Autodesk Inventor part; units mm, degrees
(part 3 of 6)
  line L865 (0, -261.6424) -> (21.9118, -283.5542) projected
  line L866 (149.4183, -199.8451) -> (131.1117, -181.5385) projected
  line L867 (131.1117, -181.5385) -> (153.0236, -159.6267) projected
  line L868 (153.0236, -159.6267) -> (165.1681, -171.7713) projected
  arc A19 (165.1681, -171.7713) -> (149.4183, -199.8451) centre (222.25, -222.25) ccw projected
  arc A20 (222.25, -146.05) -> (217.4573, -146.2009) centre (222.25, -222.25) ccw projected
  line L869 (217.4573, -146.2009) -> (229.5353, -134.1228) projected
  line L870 (229.5353, -134.1228) -> (241.4626, -146.05) projected
  line L871 (241.4626, -146.05) -> (222.25, -146.05) projected
  line L872 (280.5432, -75.9307) -> (258.6314, -54.0189) projected
  line L873 (258.6314, -54.0189) -> (280.5432, -32.1071) projected
  line L874 (280.5432, -32.1071) -> (298.45, -50.0139) projected
  line L875 (298.45, -50.0139) -> (298.45, -58.0239) projected
  line L876 (298.45, -58.0239) -> (280.5432, -75.9307) projected
  line L877 (284.1353, -28.515) -> (298.45, -14.2003) projected
  line L878 (298.45, -14.2003) -> (298.45, -42.8297) projected
  line L879 (298.45, -42.8297) -> (284.1353, -28.515) projected
  line L880 (204.0314, -57.611) -> (225.9432, -79.5228) projected
  line L881 (225.9432, -79.5228) -> (204.0314, -101.4346) projected
  line L882 (204.0314, -101.4346) -> (182.1196, -79.5228) projected
  line L883 (182.1196, -79.5228) -> (204.0314, -57.611) projected
  line L884 (102.0157, -203.4504) -> (80.1039, -181.5385) projected
  line L885 (80.1039, -181.5385) -> (102.0157, -159.6267) projected
  line L886 (102.0157, -159.6267) -> (123.9275, -181.5385) projected
  line L887 (123.9275, -181.5385) -> (102.0157, -203.4504) projected
  line L888 (36.8076, -298.45) -> (14.2003, -298.45) projected
  line L889 (14.2003, -298.45) -> (25.5039, -287.1463) projected
  line L890 (25.5039, -287.1463) -> (36.8076, -298.45) projected
  line L891 (94.9996, -298.45) -> (80.1039, -283.5542) projected
  line L892 (80.1039, -283.5542) -> (102.0157, -261.6424) projected
  line L893 (102.0157, -261.6424) -> (123.9275, -283.5542) projected
  line L894 (123.9275, -283.5542) -> (109.0318, -298.45) projected
  line L895 (109.0318, -298.45) -> (94.9996, -298.45) projected
  line L896 (-65.2081, -298.45) -> (-87.8154, -298.45) projected
  line L897 (-87.8154, -298.45) -> (-76.5118, -287.1463) projected
  line L898 (-76.5118, -287.1463) -> (-65.2081, -298.45) projected
  line L899 (-29.096, -283.5542) -> (-43.9918, -298.45) projected
  line L900 (-43.9918, -298.45) -> (-58.0239, -298.45) projected
  line L901 (-58.0239, -298.45) -> (-72.9197, -283.5542) projected
  line L902 (-72.9197, -283.5542) -> (-51.0079, -261.6424) projected
  line L903 (-51.0079, -261.6424) -> (-29.096, -283.5542) projected
  line L904 (-51.0079, -210.6346) -> (-29.096, -232.5464) projected
  line L905 (-29.096, -232.5464) -> (-51.0079, -254.4582) projected
  line L906 (-51.0079, -254.4582) -> (-72.9197, -232.5464) projected
  line L907 (-72.9197, -232.5464) -> (-51.0079, -210.6346) projected
  line L908 (-146.05, -247.4846) -> (-146.05, -222.25) projected
  arc A21 (-146.05, -222.25) -> (-146.2009, -217.4573) centre (-222.25, -222.25) ccw projected
  line L909 (-146.2009, -217.4573) -> (-131.1117, -232.5464) projected
  line L910 (-131.1117, -232.5464) -> (-146.05, -247.4846) projected
  line L911 (-51.0079, -152.4425) -> (-72.9197, -130.5307) projected
  line L912 (-72.9197, -130.5307) -> (-51.0079, -108.6189) projected
  line L913 (-51.0079, -108.6189) -> (-29.096, -130.5307) projected
  line L914 (-29.096, -130.5307) -> (-51.0079, -152.4425) projected
  line L915 (0, -101.4346) -> (-21.9118, -79.5228) projected
  line L916 (-21.9118, -79.5228) -> (0, -57.611) projected
  line L917 (0, -57.611) -> (21.9118, -79.5228) projected
  line L918 (21.9118, -79.5228) -> (0, -101.4346) projected
  line L919 (51.0079, -159.6267) -> (72.9197, -181.5385) projected
  line L920 (72.9197, -181.5385) -> (51.0079, -203.4504) projected
  line L921 (51.0079, -203.4504) -> (29.096, -181.5385) projected
  line L922 (29.096, -181.5385) -> (51.0079, -159.6267) projected
  line L923 (-76.5118, -134.1228) -> (-54.6, -156.0346) projected
  line L924 (-54.6, -156.0346) -> (-76.5118, -177.9464) projected
  line L925 (-76.5118, -177.9464) -> (-98.4236, -156.0346) projected
  line L926 (-98.4236, -156.0346) -> (-76.5118, -134.1228) projected
  line L927 (-153.0236, -108.6189) -> (-131.1117, -130.5307) projected
  line L928 (-131.1117, -130.5307) -> (-153.0236, -152.4425) projected
  line L929 (-153.0236, -152.4425) -> (-174.9354, -130.5307) projected
  line L930 (-174.9354, -130.5307) -> (-153.0236, -108.6189) projected
  line L931 (-178.5275, -83.1149) -> (-156.6157, -105.0267) projected
  line L932 (-156.6157, -105.0267) -> (-178.5275, -126.9386) projected
  line L933 (-178.5275, -126.9386) -> (-200.4393, -105.0267) projected
  line L934 (-200.4393, -105.0267) -> (-178.5275, -83.1149) projected
  line L935 (-233.1274, -79.5228) -> (-255.0393, -101.4346) projected
  line L936 (-255.0393, -101.4346) -> (-276.9511, -79.5228) projected
  line L937 (-276.9511, -79.5228) -> (-255.0393, -57.611) projected
  line L938 (-255.0393, -57.611) -> (-233.1274, -79.5228) projected
  line L939 (-258.6314, -105.0267) -> (-280.5432, -126.9386) projected
  line L940 (-280.5432, -126.9386) -> (-298.45, -109.0318) projected
  line L941 (-298.45, -109.0318) -> (-298.45, -101.0217) projected
  line L942 (-298.45, -101.0217) -> (-280.5432, -83.1149) projected
  line L943 (-280.5432, -83.1149) -> (-258.6314, -105.0267) projected
  circle A22 centre (-304.8, 0) radius 1.9939 projected
  circle A23 centre (-304.8, -44.45) radius 1.9939 projected
  circle A24 centre (-88.9, -304.8) radius 1.9939 projected
  circle A25 centre (88.9, -304.8) radius 1.9939 projected
  circle A26 centre (304.8, -44.45) radius 1.9939 projected
  circle A27 centre (304.8, 133.35) radius 1.9939 projected
  circle A28 centre (0, 304.8) radius 1.9939 projected
  circle A29 centre (-133.35, 304.8) radius 1.9939 projected
  circle A30 centre (44.45, 304.8) radius 1.9939 projected
  circle A31 centre (304.8, 88.9) radius 1.9939 projected
  circle A32 centre (304.8, -88.9) radius 1.9939 projected
  circle A33 centre (44.45, -304.8) radius 1.9939 projected
  circle A34 centre (-133.35, -304.8) radius 1.9939 projected
  circle A35 centre (-304.8, 44.45) radius 1.9939 projected
  circle A36 centre (-304.8, 133.35) radius 1.9939 projected
  circle A37 centre (-304.8, -88.9) radius 1.9939 projected
  circle A38 centre (-44.45, -304.8) radius 1.9939 projected
  circle A39 centre (133.35, -304.8) radius 1.9939 projected
  circle A40 centre (133.35, 304.8) radius 1.9939 projected
  circle A41 centre (-44.45, 304.8) radius 1.9939 projected
  circle A42 centre (-88.9, 304.8) radius 1.9939 projected
  circle A43 centre (88.9, 304.8) radius 1.9939 projected
  circle A44 centre (304.8, 44.45) radius 1.9939 projected
  circle A45 centre (304.8, -133.35) radius 1.9939 projected
  circle A46 centre (0, -304.8) radius 1.9939 projected
  circle A47 centre (-304.8, -133.35) radius 1.9939 projected
  circle A48 centre (-304.8, 88.9) radius 1.9939 projected
  line L944 (-311.15, -158.75) -> (-222.25, -158.75) projected
  arc A49 (-158.75, -222.25) -> (-222.25, -158.75) centre (-222.25, -222.25) ccw projected
  line L945 (-158.75, -222.25) -> (-158.75, -311.15) projected
  line L946 (-158.75, -311.15) -> (158.75, -311.15) projected
  line L947 (158.75, -311.15) -> (158.75, -222.25) projected
  arc A50 (222.25, -158.75) -> (158.75, -222.25) centre (222.25, -222.25) ccw projected
  line L948 (222.25, -158.75) -> (311.15, -158.75) projected
  line L949 (311.15, -158.75) -> (311.15, 158.75) projected
  line L950 (311.15, 158.75) -> (222.25, 158.75) projected
  arc A51 (158.75, 222.25) -> (222.25, 158.75) centre (222.25, 222.25) ccw projected
  line L951 (158.75, 222.25) -> (158.75, 311.15) projected
  line L952 (158.75, 311.15) -> (-158.75, 311.15) projected
  line L953 (-158.75, 311.15) -> (-158.75, 222.25) projected
  arc A52 (-222.25, 158.75) -> (-158.75, 222.25) centre (-222.25, 222.25) ccw projected
  line L954 (-222.25, 158.75) -> (-311.15, 158.75) projected
  line L955 (-311.15, 158.75) -> (-311.15, -158.75) projected
  line L956 (0, -311.15) -> (0, 311.15)
  line L957 (-311.15, 158.75) -> (-311.15, -158.75) projected
  line L958 (-311.15, 0) -> (311.15, 0)
  line L959 (81.1911, -89.119) -> (-81.1911, -89.119)
  line L960 (-81.1911, 90.2812) -> (81.1911, 90.2812)
  line L961 (84.3661, -89.119) -> (-84.3661, 90.2812) construction
  line L962 (-84.3661, -89.119) -> (84.3661, 90.2812) construction
  line L963 (88.0954, 51.4208) -> (87.5411, 51.4208)
  line L964 (73.7326, 23.3058) -> (73.7326, 21.68)
  line L965 (-84.3661, 54.5958) -> (-84.3661, 87.1062)
  line L966 (-84.3661, -85.944) -> (-84.3661, -53.4337)
  line L967 (84.3661, -53.4337) -> (84.3661, -85.944)
  line L968 (84.3661, 87.1062) -> (84.3661, 54.5958)
  arc A53 (81.1911, -89.119) -> (84.3661, -85.944) centre (81.1911, -85.944) ccw
  arc A54 (-84.3661, -85.944) -> (-81.1911, -89.119) centre (-81.1911, -85.944) ccw
  arc A55 (-81.1911, 90.2812) -> (-84.3661, 87.1062) centre (-81.1911, 87.1062) ccw
  arc A56 (84.3661, 87.1062) -> (81.1911, 90.2812) centre (81.1911, 87.1062) ccw
  arc A57 (87.5411, -50.2587) -> (84.3661, -53.4337) centre (87.5411, -53.4337) ccw
  arc A58 (84.3661, 54.5958) -> (87.5411, 51.4208) centre (87.5411, 54.5958) ccw
  line L969 (91.2704, -47.0837) -> (91.2704, 48.2458)
  line L970 (87.5411, -50.2587) -> (88.0954, -50.2587)
  line L971 (94.6634, -50.2587) -> (94.9996, -50.2587)
  arc A59 (88.0954, -50.2587) -> (91.2704, -47.0837) centre (88.0954, -47.0837) ccw
  arc A60 (91.2704, 48.2458) -> (88.0954, 51.4208) centre (88.0954, 48.2458) ccw
  line L972 (-94.6634, -50.2587) -> (-94.9996, -50.2587)
  arc A61 (-84.3661, -53.4337) -> (-87.5411, -50.2587) centre (-87.5411, -53.4337) ccw
  arc A62 (-84.3661, -53.4337) -> (-87.5411, -50.2587) centre (-87.5411, -53.4337) ccw
  arc A63 (-87.5411, 51.4208) -> (-84.3661, 54.5958) centre (-87.5411, 54.5958) ccw
  line L973 (-91.2704, -47.0837) -> (-91.2704, 48.2458)
  arc A64 (-91.2704, -47.0837) -> (-88.0954, -50.2587) centre (-88.0954, -47.0837) ccw
  arc A65 (-88.0954, 51.4208) -> (-91.2704, 48.2458) centre (-88.0954, 48.2458) ccw
  line L974 (-88.0954, -50.2587) -> (-87.5411, -50.2587)
  line L975 (-87.5411, 51.4208) -> (-88.0954, 51.4208)
  line L976 (-87.9035, -53.4337) -> (-87.9035, -85.944)
  arc A66 (-87.9035, -85.944) -> (-81.1911, -92.6564) centre (-81.1911, -85.944) ccw
  line L977 (-81.1911, -92.6564) -> (81.1911, -92.6564)
  arc A67 (81.1911, -92.6564) -> (87.9035, -85.944) centre (81.1911, -85.944) ccw
  line L978 (87.9035, -85.944) -> (87.9035, -53.7961)
  line L979 (87.9035, -53.7961) -> (88.0954, -53.7961)
  arc A68 (88.0954, -53.7961) -> (94.8078, -47.0837) centre (88.0954, -47.0837) ccw
  line L980 (94.8078, -47.0837) -> (94.8078, 48.2458)
  arc A69 (94.8078, 48.2458) -> (88.0954, 54.9582) centre (88.0954, 48.2458) ccw
  line L981 (88.0954, 54.9582) -> (87.9035, 54.9582)
  line L982 (87.9035, 54.9582) -> (87.9035, 87.1062)
  arc A70 (87.9035, 87.1062) -> (81.1911, 93.8186) centre (81.1911, 87.1062) ccw
  line L983 (81.1911, 93.8186) -> (-81.1911, 93.8186)
  arc A71 (-81.1911, 93.8186) -> (-87.9035, 87.1062) centre (-81.1911, 87.1062) ccw
  line L984 (-87.9035, 87.1062) -> (-87.9035, 54.9582)
  line L985 (-87.9035, 54.9582) -> (-88.0954, 54.9582)
  arc A72 (-88.0954, 54.9582) -> (-94.8078, 48.2458) centre (-88.0954, 48.2458) ccw
  line L986 (-94.8078, 48.2458) -> (-94.8078, -47.0837)
  arc A73 (-94.8078, -47.0837) -> (-88.0954, -53.7961) centre (-88.0954, -47.0837) ccw
  line L987 (-88.0954, -53.7961) -> (-87.5411, -53.7961)
  point P0 (0, 0)
  point P1 (84.3661, 0.5811)
  point P2 (84.3661, -50.2587)
  point P3 (-84.3661, -50.2587)
  point P4 (-84.3661, 51.4208)
  point P5 (84.3661, 51.4208)
  point P6 (-31.508, -89.119)
  point P7 (-19.4998, -89.119)
  point P8 (-84.3661, -75.2606)
  point P9 (-84.3661, -83.785)
  point P10 (-82.3116, -88.9147)
  point P11 (-70.5077, -89.119)
  point P12 (-91.2704, -17.3485)
  point P13 (-91.2704, -39.6815)
  point P14 (-91.2704, -46.8657)
  point P15 (-84.3661, -68.0764)
  point P16 (-63.3235, -89.119)
  point P17 (-38.6922, -89.119)
  point P18 (-91.2704, -10.1643)
  point P19 (-57.611, 0)
  point P20 (-44.4047, 0)
  point P21 (-6.6031, 0)
  point P22 (0, 0)
  point P23 (0, -50.4268)
  point P24 (0, -57.611)
  point P25 (0, -57.611)
  point P26 (12.3156, -89.119)
  point P27 (-12.3156, -89.119)
  point P28 (0, -89.119)
  point P29 (52.6018, 93.8186)
  point P30 (49.4139, 93.8186)
  point P31 (-87.9035, -53.7961)
  dimension "d116" = 168.7322
  dimension "d117" = 179.4002
  dimension "d120" = 3.175
  dimension "d121" = 3.175
  dimension "d122" = 3.175
  constraints: 62 end point, 42 point on circle, 21 centre point, 18 tangent, 16 point on line, 13 parallel, 13 symmetric about line, 6 equal radius, 6 midpoint, 4 horizontal, 4 perpendicular, 23 other
  measures "d116" distance of L961.end L962.end
  measures "d117" distance of L962.start L961.end
  measures "d120" radius of A53
  measures "d121" radius of A59
  measures "d122" radius of A61
extrude "Extrusion13" add sketch "Sketch12" against normal up to surface (3.175 mm away) contours L977 L183 L959 L915 | L915 L959 L956 L977 | L977 L956 L959 L918 | L918 L959 L487 L977 | L977 L186 L959 L183 | L487 L959 L488 L977 | L977 L662 L959 L186 | L488 L959 L21 L977 | L977 L663 L959 L662 | L21 L959 L24 L977 | L977 L198 L959 L663 | L24 L959 L321 L977 | L977 A66 L197 A54 L959 L198 | L321 L959 A53 L322 A67 L977 | A66 L258 L966 A54 L197 | L322 A53 L967 L832 A67 | A66 L976 L257 L966 L258 | L832 L967 L833 L978 A67 | L960 L751 L983 L956 | L956 L983 L748 L960 | L973 L187 L986 L958 | L958 L986 L188 L973 | L969 L352 L980 L958 | L958 L980 L353 L969 | L257 L976 L667 L966 | L967 L571 L978 L833 | L748 L983 L129 L960 | L960 L275 L983 L751 | L188 L986 L652 L973 | L973 L736 L986 L187 | L969 L574 L980 L352 | L353 L980 L99 L969 | L667 L976 L987 A73 L668 L973 A64 L974 A61 L966 | L967 A57 L970 A59 L969 L570 A68 L979 L978 L571 | L129 L983 L128 L960 | L960 L276 L983 L275 | L652 L986 L651 L973 | L973 L737 L986 L736 | L969 L575 L980 L574 | L99 L980 L98 L969 | L128 L983 L115 L960 | L960 L178 L983 L276 | L651 L986 L753 L973 | L973 L668 A73 L986 L737 | L969 L585 L980 L575 | L98 L980 A68 L570 L969 | L115 L983 L112 L960 | L960 L177 L983 L178 | L753 L986 A72 L985 L984 L754 L965 A63 L975 A65 L973 | L969 A60 L963 A58 L968 L584 L982 L981 A69 L980 L585 | L115 L112 L983 | L112 L983 L822 L960 | L960 L165 L983 L177 | L822 L983 A70 L821 L968 A56 L960 | L960 A55 L965 L166 A71 L983 L165 | L984 L172 L965 L754 | L584 L968 L350 L982 | L821 A70 L982 L351 L968 | L965 L171 L984 A71 L166 | L984 L171 L965 L172 | L350 L968 L351 L982
sketch "Sketch13" plane through (0, 3.175, 0) normal (0, 1, 0) x (1, 0, 0)
  line L0 (-70.5077, -89.119) -> (-81.1911, -89.119) projected
  arc A0 (-82.3116, -88.9147) -> (-81.1911, -89.119) centre (-81.1911, -85.944) ccw projected
  line L1 (-84.3661, -83.785) -> (-84.3661, -75.2606) projected
  line L2 (81.1911, -89.119) -> (70.5077, -89.119) projected
  line L3 (84.3661, -75.2606) -> (84.3661, -83.785) projected
  line L4 (-78.0506, -89.119) -> (-81.1911, -89.119)
  line L5 (-84.3661, -80.2772) -> (-84.3661, -85.944)
  line L6 (63.3235, 90.2812) -> (81.1911, 90.2812) projected
  line L7 (84.3661, 77.763) -> (84.3661, 69.2385) projected
  line L8 (84.3661, 87.1062) -> (84.3661, 84.9472) projected
  line L9 (78.1452, 90.2812) -> (81.1911, 90.2812)
  line L10 (84.3661, 87.1062) -> (84.3661, 85.7634)
  line L11 (81.1911, 90.2812) -> (-81.1911, 90.2812)
  line L12 (-81.1911, -89.119) -> (81.1911, -89.119)
  arc A1 (-84.3661, -85.944) -> (-81.1911, -89.119) centre (-81.1911, -85.944) ccw
  arc A2 (81.1911, -89.119) -> (84.3661, -85.944) centre (81.1911, -85.944) ccw
  arc A3 (-84.3661, -85.944) -> (-81.1911, -89.119) centre (-81.1911, -85.944) ccw
  arc A4 (-81.1911, 90.2812) -> (-84.3661, 87.1062) centre (-81.1911, 87.1062) ccw
  arc A5 (84.3661, 87.1062) -> (81.1911, 90.2812) centre (81.1911, 87.1062) ccw
  arc A6 (84.3661, 87.1062) -> (81.1911, 90.2812) centre (81.1911, 87.1062) ccw
  arc A7 (87.5411, -50.2587) -> (84.3661, -53.4337) centre (87.5411, -53.4337) ccw projected
  arc A8 (88.0954, -50.2587) -> (91.2704, -47.0837) centre (88.0954, -47.0837) ccw projected
  line L13 (91.2704, -17.3485) -> (91.2704, -39.6815) projected
  arc A9 (84.3661, 54.5958) -> (87.5411, 51.4208) centre (87.5411, 54.5958) ccw projected
  arc A10 (91.2704, 48.2458) -> (88.0954, 51.4208) centre (88.0954, 48.2458) ccw projected
  line L14 (91.2704, 48.2458) -> (91.2704, 40.8436) projected
  line L15 (91.2704, -39.6815) -> (91.2704, -17.3485) projected
  line L16 (84.3661, -85.944) -> (84.3661, -53.4337)
  line L17 (84.3661, 54.5958) -> (84.3661, 87.1062)
  arc A11 (-84.3661, -53.4337) -> (-87.5411, -50.2587) centre (-87.5411, -53.4337) ccw projected
  arc A12 (-91.2704, -47.0837) -> (-88.0954, -50.2587) centre (-88.0954, -47.0837) ccw projected
  line L18 (-87.5411, -50.2587) -> (-88.0954, -50.2587) projected
  line L19 (-91.2704, -47.0837) -> (-91.2704, -46.8657) projected
  arc A13 (-87.5411, 51.4208) -> (-84.3661, 54.5958) centre (-87.5411, 54.5958) ccw projected
  arc A14 (-88.0954, 51.4208) -> (-91.2704, 48.2458) centre (-88.0954, 48.2458) ccw projected
  line L20 (-91.2704, 40.8436) -> (-91.2704, 48.2458) projected
  line L21 (-91.2704, -46.8657) -> (-91.2704, 40.8436)
  line L22 (-84.3661, 87.1062) -> (-84.3661, 54.5958)
  line L23 (-84.3661, -53.4337) -> (-84.3661, -85.944)
  line L24 (91.2704, -46.8657) -> (91.2704, -47.0837) projected
  line L25 (91.2704, 40.8436) -> (91.2704, 48.2458) projected
  line L26 (91.2704, 44.2779) -> (91.2704, -46.8657)
  line L27 (87.5411, 51.4208) -> (88.0954, 51.4208) projected
  line L28 (88.0954, -50.2587) -> (87.5411, -50.2587) projected
  line L29 (-88.0954, 51.4208) -> (-87.5411, 51.4208) projected
  point P0 (0, 0)
  point P1 (-85.248, -89.119)
  point P2 (-84.3661, -89.119)
  point P3 (84.3661, 90.2812)
  point P4 (-82.3116, -88.9147)
  dimension "d125" = 3.175
  constraints: 24 end point, 16 point on circle, 16 tangent, 15 point on line, 6 centre point, 5 equal radius, 5 parallel, 2 collinear, 2 perpendicular, 1 horizontal
  measures "d125" radius of A1
extrude "Extrusion14" cut sketch "Sketch13" against normal blind 80.9625
sketch "Sketch14" plane through (0, 3.175, 0) normal (0, 1, 0) x (1, 0, 0)
  arc A0 (-84.9214, -91.5245) -> (-81.1911, -92.6564) centre (-81.1911, -85.944) ccw projected
  line L0 (-81.1911, -92.6564) -> (-66.9703, -92.6564) projected
  line L1 (-79.3946, -92.6564) -> (-81.1979, -92.6564)
  line L2 (-81.1911, 90.2812) -> (81.1911, 90.2812) projected
  line L3 (87.9035, 65.7011) -> (87.9035, 81.3004) projected
  line L4 (81.1911, 93.8186) -> (59.7861, 93.8186) projected
  line L5 (87.9035, 76.3407) -> (87.9035, 87.113)
  line L6 (81.1979, 93.8186) -> (78.2104, 93.8186)
  line L7 (-81.1979, -92.6564) -> (81.1979, -92.6564)
  line L8 (81.1979, 93.8186) -> (-81.1979, 93.8186)
  line L9 (-87.9035, 87.113) -> (-87.9035, 54.9582)
  line L10 (-94.8078, -13.8111) -> (-94.8078, -43.2189) projected
  line L11 (-94.8078, -41.8566) -> (-94.8078, -47.0905)
  line L12 (-88.1022, -53.7961) -> (-88.0954, -53.7961)
  arc A1 (-94.2247, -49.82) -> (-88.0954, -53.7961) centre (-88.0954, -47.0837) ccw projected
  arc A2 (-94.8078, -47.0905) -> (-88.1022, -53.7961) centre (-88.1022, -47.0905) ccw
  arc A3 (-88.0954, 54.9582) -> (-94.8078, 48.2458) centre (-88.0954, 48.2458) ccw projected
  line L13 (-87.9035, 54.9582) -> (-88.0954, 54.9582) projected
  line L14 (-94.8078, 48.2458) -> (-94.8078, 44.381) projected
  line L15 (-94.8078, 46.3134) -> (-94.8078, -47.0905)
  arc A4 (-87.9035, -85.9508) -> (-81.1979, -92.6564) centre (-81.1979, -85.9508) ccw
  arc A5 (-81.1979, 93.8186) -> (-87.9035, 87.113) centre (-81.1979, 87.113) ccw
  arc A6 (87.9035, 87.113) -> (81.1979, 93.8186) centre (81.1979, 87.113) ccw
  line L16 (87.9035, -85.9508) -> (87.9035, -53.7961)
  line L17 (87.9035, 54.9582) -> (87.9035, 87.113)
  line L18 (94.8078, -43.2189) -> (94.8078, -13.8111) projected
  line L19 (94.8078, 44.381) -> (94.8078, 48.2458) projected
  arc A7 (94.8078, 48.2458) -> (88.0954, 54.9582) centre (88.0954, 48.2458) ccw projected
  line L20 (88.0954, 54.9582) -> (87.9035, 54.9582) projected
  arc A8 (88.0954, -53.7961) -> (94.2247, -49.82) centre (88.0954, -47.0837) ccw projected
  line L21 (87.9035, -53.7961) -> (88.0954, -53.7961) projected
  line L22 (94.8078, 46.3134) -> (94.8078, -47.0905)
  line L23 (88.1022, -53.7961) -> (88.0954, -53.7961)
  arc A9 (88.1022, -53.7961) -> (94.8078, -47.0905) centre (88.1022, -47.0905) ccw
  arc A10 (81.1979, -92.6564) -> (87.9035, -85.9508) centre (81.1979, -85.9508) ccw
  line L24 (81.1979, -92.6564) -> (-81.1979, -92.6564)
  line L25 (-87.9035, -85.9508) -> (-87.9035, -53.7961)
  line L26 (-94.8078, -47.0905) -> (-94.8078, 46.3134)
  line L27 (-87.9035, 58.5169) -> (-87.9035, 54.9582) projected
  line L28 (-87.9035, 54.9582) -> (-87.9035, 87.113)
  line L29 (-81.1979, 93.8186) -> (81.1979, 93.8186)
  line L30 (87.9035, 87.113) -> (87.9035, 54.9582)
  line L31 (-81.1979, -102.0798) -> (81.1979, -102.0798)
  arc A11 (-97.3269, -85.9508) -> (-81.1979, -102.0798) centre (-81.1979, -85.9508) ccw
  line L32 (-88.0954, -53.7961) -> (-87.9035, -53.7961) projected
  line L33 (-87.9035, -53.7961) -> (-88.0954, -53.7961)
  line L34 (97.325, -60.3125) -> (97.325, -85.9508)
  arc A12 (81.1979, -102.0779) -> (97.325, -85.9508) centre (81.1979, -85.9508) ccw
  line L35 (104.223, 44.3468) -> (104.223, -47.0905)
  arc A13 (97.325, -60.3125) -> (104.223, -47.0905) centre (88.1022, -47.0905) ccw
  line L36 (88.1022, -63.2113) -> (88.0954, -63.2113)
  line L37 (87.9035, 64.3816) -> (88.0954, 64.3816)
  arc A14 (104.2312, 48.2458) -> (97.3269, 61.4799) centre (88.0954, 48.2458) ccw
  line L38 (104.2312, 48.2458) -> (104.2312, 44.381)
  line L39 (97.3269, 61.4799) -> (97.3269, 87.113)
  arc A15 (97.3269, 87.113) -> (81.1979, 103.242) centre (81.1979, 87.113) ccw
  line L40 (81.1979, 103.242) -> (-81.1979, 103.242)
  arc A16 (-81.1979, 103.242) -> (-97.3269, 87.113) centre (-81.1979, 87.113) ccw
  line L41 (-97.3269, 87.113) -> (-97.3269, 61.4799)
  line L42 (-94.8078, -47.0905) -> (-94.8078, 46.3134)
  line L43 (-104.2312, -47.0905) -> (-104.2312, 46.3134)
  line L44 (-104.2312, 46.3134) -> (-104.2312, 48.2458)
  arc A17 (-94.8078, -47.0905) -> (-88.0988, -53.7961) centre (-88.1022, -47.0905) ccw
  arc A18 (-104.2312, -47.0905) -> (-97.3269, -60.3211) centre (-88.1022, -47.0905) ccw
  line L45 (-97.3269, -85.9508) -> (-97.3269, -60.3211)
  arc A19 (-97.3269, 61.4799) -> (-104.2312, 48.2458) centre (-88.0954, 48.2458) ccw
  arc A20 (87.5411, -50.2587) -> (84.3661, -53.4337) centre (87.5411, -53.4337) ccw projected
  line L46 (88.0954, -50.2587) -> (87.5411, -50.2587) projected
  line L47 (88.0954, -53.7961) -> (87.9035, -53.7961) projected
  line L48 (87.5411, -50.2587) -> (88.0954, -50.2587) projected
  arc A21 (87.5411, -50.2587) -> (84.3661, -53.4337) centre (87.5411, -53.4337) ccw projected
  line L49 (102.0157, 51.5889) -> (87.9035, 65.7011) projected
  line L50 (87.9035, 58.5169) -> (98.4236, 47.9968) projected
  line L51 (87.9035, 54.9582) -> (87.9035, 58.5169) projected
  line L52 (87.9035, 54.9582) -> (88.0954, 54.9582) projected
  line L53 (87.9035, 58.5169) -> (87.9035, 54.9582) projected
  line L54 (98.4236, 47.9968) -> (87.9035, 58.5169) projected
  line L55 (87.9035, 65.7011) -> (102.0157, 51.5889) projected
  line L56 (98.4236, 47.9968) -> (87.9035, 58.5169) projected
  line L57 (87.9035, 58.5169) -> (98.4236, 47.9968) projected
  line L58 (87.5411, 51.4208) -> (88.0954, 51.4208) projected
  arc A22 (84.3661, 54.5958) -> (87.5411, 51.4208) centre (87.5411, 54.5958) ccw projected
  arc A23 (84.3661, 54.5958) -> (87.5411, 51.4208) centre (87.5411, 54.5958) ccw projected
  line L59 (88.0954, 51.4208) -> (87.5411, 51.4208) projected
  line L60 (88.0954, 51.4208) -> (87.5411, 51.4208) projected
  line L61 (87.5411, 51.4208) -> (88.0954, 51.4208) projected
  arc A24 (84.3661, 54.5958) -> (87.5411, 51.4208) centre (87.5411, 54.5958) ccw projected
  arc A25 (84.3661, 54.5958) -> (87.5411, 51.4208) centre (87.5411, 54.5958) ccw projected
  line L62 (66.9703, -92.6564) -> (81.1911, -92.6564) projected
  line L63 (81.1911, -92.6564) -> (66.9703, -92.6564) projected
  line L64 (54.6, -105.0267) -> (66.9703, -92.6564) projected
  line L65 (66.9703, -92.6564) -> (54.6, -105.0267) projected
  line L66 (59.7861, -92.6564) -> (51.0079, -101.4346) projected
  line L67 (51.0079, -101.4346) -> (59.7861, -92.6564) projected
  arc A26 (81.1911, -92.6564) -> (84.9214, -91.5245) centre (81.1911, -85.944) ccw projected
  arc A27 (81.1911, -92.6564) -> (84.9214, -91.5245) centre (81.1911, -85.944) ccw projected
  line L68 (84.9214, -91.5245) -> (98.4236, -105.0267) projected
  line L69 (98.4236, -105.0267) -> (84.9214, -91.5245) projected
  line L70 (102.0157, -101.4346) -> (87.7843, -87.2033) projected
  line L71 (87.7843, -87.2033) -> (102.0157, -101.4346) projected
  line L72 (98.4236, -54.0189) -> (87.9035, -64.539) projected
  line L73 (87.9035, -64.539) -> (87.9035, -53.7961) projected
  line L74 (87.9035, -71.7232) -> (102.0157, -57.611) projected
  line L75 (87.9035, -85.944) -> (87.9035, -71.7232) projected
  arc A28 (87.7843, -87.2033) -> (87.9035, -85.944) centre (81.1911, -85.944) ccw projected
  arc A29 (81.1911, -89.119) -> (84.3661, -85.944) centre (81.1911, -85.944) ccw projected
  line L76 (84.3661, -53.4337) -> (84.3661, -85.944) projected
  arc A30 (87.7843, -87.2033) -> (87.9035, -85.944) centre (81.1911, -85.944) ccw projected
  line L77 (87.9035, -71.7232) -> (87.9035, -85.944) projected
  line L78 (102.0157, -57.611) -> (87.9035, -71.7232) projected
  line L79 (87.9035, -53.7961) -> (87.9035, -64.539) projected
  line L80 (87.9035, -64.539) -> (98.4236, -54.0189) projected
  line L81 (84.3661, -85.944) -> (84.3661, -53.4337) projected
  arc A31 (81.1911, -89.119) -> (84.3661, -85.944) centre (81.1911, -85.944) ccw projected
  line L82 (84.3661, -53.4337) -> (84.3661, -85.944) projected
  line L83 (84.3661, -85.944) -> (84.3661, -53.4337) projected
  arc A32 (81.1911, -89.119) -> (84.3661, -85.944) centre (81.1911, -85.944) ccw projected
  arc A33 (81.1911, -89.119) -> (84.3661, -85.944) centre (81.1911, -85.944) ccw projected
  line L84 (88.0954, -53.7961) -> (87.9035, -53.7961) projected
  line L85 (87.9035, -53.7961) -> (88.0954, -53.7961) projected
  arc A34 (87.5411, -50.2587) -> (84.3661, -53.4337) centre (87.5411, -53.4337) ccw projected
  arc A35 (87.5411, -50.2587) -> (84.3661, -53.4337) centre (87.5411, -53.4337) ccw projected
  line L86 (87.5411, -50.2587) -> (88.0954, -50.2587) projected
  line L87 (88.0954, -50.2587) -> (87.5411, -50.2587) projected
  line L88 (98.4236, 99.0047) -> (87.7843, 88.3654) projected
  line L89 (87.7843, 88.3654) -> (98.4236, 99.0047) projected
  line L90 (87.9035, 81.3004) -> (102.0157, 95.4126) projected
  line L91 (102.0157, 95.4126) -> (87.9035, 81.3004) projected
  arc A36 (87.7843, 88.3654) -> (81.1911, 93.8186) centre (81.1911, 87.1062) ccw projected
  arc A37 (87.7843, 88.3654) -> (81.1911, 93.8186) centre (81.1911, 87.1062) ccw projected
  arc A38 (84.3661, 87.1062) -> (81.1911, 90.2812) centre (81.1911, 87.1062) ccw projected
  arc A39 (84.3661, 87.1062) -> (81.1911, 90.2812) centre (81.1911, 87.1062) ccw projected
  line L92 (47.4158, 99.0047) -> (42.2297, 93.8186) projected
  line L93 (59.7861, 93.8186) -> (54.6, 99.0047) projected
  line L94 (59.7861, 93.8186) -> (81.1911, 93.8186) projected
  line L95 (54.6, 99.0047) -> (59.7861, 93.8186) projected
  line L96 (42.2297, 93.8186) -> (47.4158, 99.0047) projected
  line L97 (84.3661, 87.1062) -> (84.3661, 54.5958) projected
  line L98 (87.9035, 81.3004) -> (87.9035, 65.7011) projected
  line L99 (84.3661, 54.5958) -> (84.3661, 87.1062) projected
  line L100 (84.3661, 87.1062) -> (84.3661, 54.5958) projected
  line L101 (84.3661, 54.5958) -> (84.3661, 87.1062) projected
  arc A40 (87.7843, -87.2033) -> (87.9035, -85.944) centre (81.1911, -85.944) ccw projected
  arc A41 (87.7843, -87.2033) -> (87.9035, -85.944) centre (81.1911, -85.944) ccw projected
  line L102 (87.9035, -85.944) -> (87.9035, -71.7232) projected
  line L103 (87.9035, -71.7232) -> (87.9035, -85.944) projected
  line L104 (87.9035, -53.7961) -> (87.9035, -64.539) projected
  line L105 (87.9035, -64.539) -> (87.9035, -53.7961) projected
  line L106 (42.2297, -92.6564) -> (59.7861, -92.6564) projected
  line L107 (51.0079, -101.4346) -> (42.2297, -92.6564) projected
  line L108 (42.2297, -92.6564) -> (51.0079, -101.4346) projected
  line L109 (59.7861, -92.6564) -> (42.2297, -92.6564) projected
  line L110 (42.2297, -92.6564) -> (59.7861, -92.6564) projected
  line L111 (59.7861, -92.6564) -> (42.2297, -92.6564) projected
  line L112 (51.0079, -101.4346) -> (59.7861, -92.6564) projected
  line L113 (59.7861, -92.6564) -> (51.0079, -101.4346) projected
  line L114 (54.6, -105.0267) -> (66.9703, -92.6564) projected
  line L115 (66.9703, -92.6564) -> (54.6, -105.0267) projected
  line L116 (81.1911, -92.6564) -> (66.9703, -92.6564) projected
  line L117 (66.9703, -92.6564) -> (81.1911, -92.6564) projected
  arc A42 (81.1911, -92.6564) -> (84.9214, -91.5245) centre (81.1911, -85.944) ccw projected
  arc A43 (81.1911, -92.6564) -> (84.9214, -91.5245) centre (81.1911, -85.944) ccw projected
  line L118 (98.4236, -105.0267) -> (84.9214, -91.5245) projected
  line L119 (84.9214, -91.5245) -> (98.4236, -105.0267) projected
  line L120 (102.0157, -101.4346) -> (87.7843, -87.2033) projected
  line L121 (87.7843, -87.2033) -> (102.0157, -101.4346) projected
  line L122 (15.9624, -92.6564) -> (35.0455, -92.6564) projected
  line L123 (3.5921, -105.0267) -> (15.9624, -92.6564) projected
  line L124 (35.0455, -92.6564) -> (47.4158, -105.0267) projected
  line L125 (47.4158, -105.0267) -> (35.0455, -92.6564) projected
  line L126 (15.9624, -92.6564) -> (3.5921, -105.0267) projected
  line L127 (35.0455, -92.6564) -> (15.9624, -92.6564) projected
  line L128 (98.4236, -54.0189) -> (87.9035, -64.539) projected
  line L129 (87.9035, -64.539) -> (98.4236, -54.0189) projected
  line L130 (102.0157, -57.611) -> (87.9035, -71.7232) projected
  line L131 (87.9035, -71.7232) -> (102.0157, -57.611) projected
  line L132 (-88.0954, 51.4208) -> (-87.5411, 51.4208) projected
  line L133 (-87.5411, 51.4208) -> (-88.0954, 51.4208) projected
  line L134 (-87.5411, 51.4208) -> (-88.0954, 51.4208) projected
  line L135 (-88.0954, 51.4208) -> (-87.5411, 51.4208) projected
  arc A44 (-87.5411, 51.4208) -> (-84.3661, 54.5958) centre (-87.5411, 54.5958) ccw projected
  arc A45 (-87.5411, 51.4208) -> (-84.3661, 54.5958) centre (-87.5411, 54.5958) ccw projected
  arc A46 (-87.5411, 51.4208) -> (-84.3661, 54.5958) centre (-87.5411, 54.5958) ccw projected
  arc A47 (-87.5411, 51.4208) -> (-84.3661, 54.5958) centre (-87.5411, 54.5958) ccw projected
  line L136 (-87.5411, -50.2587) -> (-88.0954, -50.2587) projected
  line L137 (-88.0954, -50.2587) -> (-87.5411, -50.2587) projected
  line L138 (-88.0954, -50.2587) -> (-87.5411, -50.2587) projected
  line L139 (-87.5411, -50.2587) -> (-88.0954, -50.2587) projected
  arc A48 (-84.3661, -53.4337) -> (-87.5411, -50.2587) centre (-87.5411, -53.4337) ccw projected
  arc A49 (-84.3661, -53.4337) -> (-87.5411, -50.2587) centre (-87.5411, -53.4337) ccw projected
  arc A50 (-84.3661, -53.4337) -> (-87.5411, -50.2587) centre (-87.5411, -53.4337) ccw projected
  arc A51 (-84.3661, -53.4337) -> (-87.5411, -50.2587) centre (-87.5411, -53.4337) ccw projected
  line L140 (-35.0455, -92.6564) -> (-15.9624, -92.6564) projected
  line L141 (-15.9624, -92.6564) -> (-35.0455, -92.6564) projected
  line L142 (-15.9624, -92.6564) -> (-35.0455, -92.6564) projected
  line L143 (-35.0455, -92.6564) -> (-15.9624, -92.6564) projected
  line L144 (0, -101.4346) -> (-8.7782, -92.6564) projected
  line L145 (-15.9624, -92.6564) -> (-3.5921, -105.0267) projected
  line L146 (-3.5921, -105.0267) -> (-15.9624, -92.6564) projected
  line L147 (-8.7782, -92.6564) -> (0, -101.4346) projected
  line L148 (0, -101.4346) -> (-8.7782, -92.6564) projected
  line L149 (-8.7782, -92.6564) -> (0, -101.4346) projected
  line L150 (-3.5921, -105.0267) -> (-15.9624, -92.6564) projected
  line L151 (-15.9624, -92.6564) -> (-3.5921, -105.0267) projected
  line L152 (-42.2297, 93.8186) -> (-47.4158, 99.0047) projected
  line L153 (-47.4158, 99.0047) -> (-42.2297, 93.8186) projected
  line L154 (-8.7782, 93.8186) -> (-42.2297, 93.8186) projected
  line L155 (-42.2297, 93.8186) -> (-8.7782, 93.8186) projected
  line L156 (-8.7782, 93.8186) -> (-42.2297, 93.8186) projected
  line L157 (-42.2297, 93.8186) -> (-8.7782, 93.8186) projected
  line L158 (-3.5921, 99.0047) -> (-8.7782, 93.8186) projected
  line L159 (-8.7782, 93.8186) -> (-3.5921, 99.0047) projected
  line L160 (-3.5921, 99.0047) -> (-8.7782, 93.8186) projected
  line L161 (-8.7782, 93.8186) -> (-3.5921, 99.0047) projected
  line L162 (-1.594, 93.8186) -> (0, 95.4126) projected
  line L163 (0, 95.4126) -> (-1.594, 93.8186) projected
  line L164 (-54.6, 99.0047) -> (-59.7861, 93.8186) projected
  line L165 (-59.7861, 93.8186) -> (-54.6, 99.0047) projected
  line L166 (-52.6018, 93.8186) -> (-51.0079, 95.4126) projected
  line L167 (-51.0079, 95.4126) -> (-52.6018, 93.8186) projected
  line L168 (-59.7861, 93.8186) -> (-81.1911, 93.8186) projected
  arc A52 (-81.1911, 90.2812) -> (-84.3661, 87.1062) centre (-81.1911, 87.1062) ccw projected
  arc A53 (-81.1911, 90.2812) -> (-84.3661, 87.1062) centre (-81.1911, 87.1062) ccw projected
  line L169 (-81.1911, 93.8186) -> (-59.7861, 93.8186) projected
  arc A54 (-81.1911, 90.2812) -> (-84.3661, 87.1062) centre (-81.1911, 87.1062) ccw projected
  arc A55 (-81.1911, 90.2812) -> (-84.3661, 87.1062) centre (-81.1911, 87.1062) ccw projected
  line L170 (-81.1911, 93.8186) -> (-59.7861, 93.8186) projected
  line L171 (-59.7861, 93.8186) -> (-81.1911, 93.8186) projected
  line L172 (-87.7843, 88.3654) -> (-98.4236, 99.0047) projected
  line L173 (-84.3661, 54.5958) -> (-84.3661, 87.1062) projected
  line L174 (-84.3661, 87.1062) -> (-84.3661, 54.5958) projected
  line L175 (-98.4236, 99.0047) -> (-87.7843, 88.3654) projected
  line L176 (-84.3661, 87.1062) -> (-84.3661, 54.5958) projected
  line L177 (-84.3661, 54.5958) -> (-84.3661, 87.1062) projected
  line L178 (0, 95.4126) -> (1.594, 93.8186) projected
  line L179 (1.594, 93.8186) -> (-1.594, 93.8186) projected
  line L180 (8.7782, 93.8186) -> (3.5921, 99.0047) projected
  line L181 (3.5921, 99.0047) -> (8.7782, 93.8186) projected
  line L182 (-1.594, 93.8186) -> (1.594, 93.8186) projected
  line L183 (1.594, 93.8186) -> (0, 95.4126) projected
  line L184 (0, 95.4126) -> (-1.594, 93.8186) projected
  line L185 (-1.594, 93.8186) -> (0, 95.4126) projected
  line L186 (-1.594, 93.8186) -> (1.594, 93.8186) projected
  line L187 (1.594, 93.8186) -> (-1.594, 93.8186) projected
  line L188 (0, 95.4126) -> (1.594, 93.8186) projected
  line L189 (1.594, 93.8186) -> (0, 95.4126) projected
  line L190 (3.5921, 99.0047) -> (8.7782, 93.8186) projected
  line L191 (8.7782, 93.8186) -> (3.5921, 99.0047) projected
  arc A56 (-81.1911, 93.8186) -> (-87.7843, 88.3654) centre (-81.1911, 87.1062) ccw projected
  arc A57 (-81.1911, 93.8186) -> (-87.7843, 88.3654) centre (-81.1911, 87.1062) ccw projected
  arc A58 (-81.1911, 93.8186) -> (-87.7843, 88.3654) centre (-81.1911, 87.1062) ccw projected
  arc A59 (-81.1911, 93.8186) -> (-87.7843, 88.3654) centre (-81.1911, 87.1062) ccw projected
  line L192 (-98.4236, 99.0047) -> (-87.7843, 88.3654) projected
  line L193 (-87.7843, 88.3654) -> (-98.4236, 99.0047) projected
  line L194 (-49.4139, 93.8186) -> (-52.6018, 93.8186) projected
  line L195 (-51.0079, 95.4126) -> (-49.4139, 93.8186) projected
  line L196 (-49.4139, 93.8186) -> (-51.0079, 95.4126) projected
  line L197 (-52.6018, 93.8186) -> (-49.4139, 93.8186) projected
  line L198 (-47.4158, 99.0047) -> (-42.2297, 93.8186) projected
  line L199 (-42.2297, 93.8186) -> (-47.4158, 99.0047) projected
  line L200 (-51.0079, 95.4126) -> (-49.4139, 93.8186) projected
  line L201 (-49.4139, 93.8186) -> (-51.0079, 95.4126) projected
  line L202 (-51.0079, 95.4126) -> (-52.6018, 93.8186) projected
  line L203 (-52.6018, 93.8186) -> (-51.0079, 95.4126) projected
  line L204 (-49.4139, 93.8186) -> (-52.6018, 93.8186) projected
  line L205 (-52.6018, 93.8186) -> (-49.4139, 93.8186) projected
  line L206 (-54.6, 99.0047) -> (-59.7861, 93.8186) projected
  line L207 (-59.7861, 93.8186) -> (-54.6, 99.0047) projected
  arc A60 (-84.9214, -91.5245) -> (-81.1911, -92.6564) centre (-81.1911, -85.944) ccw projected
  arc A61 (-84.9214, -91.5245) -> (-81.1911, -92.6564) centre (-81.1911, -85.944) ccw projected
  arc A62 (-84.9214, -91.5245) -> (-81.1911, -92.6564) centre (-81.1911, -85.944) ccw projected
  line L208 (-98.4236, -105.0267) -> (-84.9214, -91.5245) projected
  line L209 (-84.9214, -91.5245) -> (-98.4236, -105.0267) projected
  line L210 (-98.4236, -105.0267) -> (-84.9214, -91.5245) projected
  line L211 (-84.9214, -91.5245) -> (-98.4236, -105.0267) projected
  arc A63 (-84.3661, -85.944) -> (-81.1911, -89.119) centre (-81.1911, -85.944) ccw projected
  arc A64 (-84.3661, -85.944) -> (-81.1911, -89.119) centre (-81.1911, -85.944) ccw projected
  arc A65 (-84.3661, -85.944) -> (-81.1911, -89.119) centre (-81.1911, -85.944) ccw projected
  arc A66 (-84.3661, -85.944) -> (-81.1911, -89.119) centre (-81.1911, -85.944) ccw projected
  line L212 (-87.7843, -87.2033) -> (-102.0157, -101.4346) projected
  line L213 (-102.0157, -101.4346) -> (-87.7843, -87.2033) projected
  line L214 (-102.0157, -101.4346) -> (-87.7843, -87.2033) projected
  line L215 (-87.7843, -87.2033) -> (-102.0157, -101.4346) projected
  arc A67 (-87.9035, -85.944) -> (-87.7843, -87.2033) centre (-81.1911, -85.944) ccw projected
  arc A68 (-87.9035, -85.944) -> (-87.7843, -87.2033) centre (-81.1911, -85.944) ccw projected
  arc A69 (-87.9035, -85.944) -> (-87.7843, -87.2033) centre (-81.1911, -85.944) ccw projected
  line L216 (-47.4158, -105.0267) -> (-35.0455, -92.6564) projected
  line L217 (-51.0079, -101.4346) -> (-59.7861, -92.6564) projected
  line L218 (-42.2297, -92.6564) -> (-51.0079, -101.4346) projected
  line L219 (-59.7861, -92.6564) -> (-42.2297, -92.6564) projected
  line L220 (-42.2297, -92.6564) -> (-59.7861, -92.6564) projected
  line L221 (-51.0079, -101.4346) -> (-42.2297, -92.6564) projected
  line L222 (-59.7861, -92.6564) -> (-51.0079, -101.4346) projected
  line L223 (-35.0455, -92.6564) -> (-47.4158, -105.0267) projected
  line L224 (-66.9703, -92.6564) -> (-81.1911, -92.6564) projected
  line L225 (-66.9703, -92.6564) -> (-54.6, -105.0267) projected
  line L226 (-54.6, -105.0267) -> (-66.9703, -92.6564) projected
  line L227 (-81.1911, -92.6564) -> (-66.9703, -92.6564) projected
  line L228 (-66.9703, -92.6564) -> (-81.1911, -92.6564) projected
  line L229 (-54.6, -105.0267) -> (-66.9703, -92.6564) projected
  line L230 (-66.9703, -92.6564) -> (-54.6, -105.0267) projected
  line L231 (-51.0079, -101.4346) -> (-42.2297, -92.6564) projected
  line L232 (-42.2297, -92.6564) -> (-51.0079, -101.4346) projected
  line L233 (8.7782, -92.6564) -> (0, -101.4346) projected
  line L234 (-8.7782, -92.6564) -> (8.7782, -92.6564) projected
  line L235 (8.7782, -92.6564) -> (-8.7782, -92.6564) projected
  line L236 (0, -101.4346) -> (8.7782, -92.6564) projected
  line L237 (8.7782, -92.6564) -> (-8.7782, -92.6564) projected
  line L238 (-8.7782, -92.6564) -> (8.7782, -92.6564) projected
  line L239 (0, -101.4346) -> (8.7782, -92.6564) projected
  line L240 (8.7782, -92.6564) -> (0, -101.4346) projected
  line L241 (3.5921, -105.0267) -> (15.9624, -92.6564) projected
  line L242 (15.9624, -92.6564) -> (3.5921, -105.0267) projected
  line L243 (-42.2297, -92.6564) -> (-59.7861, -92.6564) projected
  line L244 (-59.7861, -92.6564) -> (-42.2297, -92.6564) projected
  line L245 (-51.0079, -101.4346) -> (-59.7861, -92.6564) projected
  line L246 (-59.7861, -92.6564) -> (-51.0079, -101.4346) projected
  line L247 (-47.4158, -105.0267) -> (-35.0455, -92.6564) projected
  line L248 (-35.0455, -92.6564) -> (-47.4158, -105.0267) projected
  line L249 (15.9624, -92.6564) -> (35.0455, -92.6564) projected
  line L250 (35.0455, -92.6564) -> (15.9624, -92.6564) projected
  line L251 (42.2297, 93.8186) -> (8.7782, 93.8186) projected
  line L252 (8.7782, 93.8186) -> (42.2297, 93.8186) projected
  line L253 (81.1911, 90.2812) -> (-81.1911, 90.2812) projected
  line L254 (-81.1911, 90.2812) -> (81.1911, 90.2812) projected
  line L255 (81.1911, 90.2812) -> (-81.1911, 90.2812) projected
  line L256 (47.4158, 99.0047) -> (42.2297, 93.8186) projected
  line L257 (42.2297, 93.8186) -> (47.4158, 99.0047) projected
  line L258 (8.7782, 93.8186) -> (42.2297, 93.8186) projected
  line L259 (42.2297, 93.8186) -> (8.7782, 93.8186) projected
  line L260 (102.0157, 51.5889) -> (87.9035, 65.7011) projected
  line L261 (87.9035, 65.7011) -> (102.0157, 51.5889) projected
  line L262 (87.9035, 54.9582) -> (88.0954, 54.9582) projected
  line L263 (88.0954, 54.9582) -> (87.9035, 54.9582) projected
  line L264 (87.9035, 54.9582) -> (87.9035, 58.5169) projected
  line L265 (87.9035, 58.5169) -> (87.9035, 54.9582) projected
  line L266 (87.9035, 81.3004) -> (87.9035, 65.7011) projected
  line L267 (87.9035, 65.7011) -> (87.9035, 81.3004) projected
  arc A70 (84.3661, 87.1062) -> (81.1911, 90.2812) centre (81.1911, 87.1062) ccw projected
  arc A71 (84.3661, 87.1062) -> (81.1911, 90.2812) centre (81.1911, 87.1062) ccw projected
  arc A72 (87.7843, 88.3654) -> (81.1911, 93.8186) centre (81.1911, 87.1062) ccw projected
  arc A73 (87.7843, 88.3654) -> (81.1911, 93.8186) centre (81.1911, 87.1062) ccw projected
  line L268 (102.0157, 95.4126) -> (87.9035, 81.3004) projected
  line L269 (87.9035, 81.3004) -> (102.0157, 95.4126) projected
  line L270 (98.4236, 99.0047) -> (87.7843, 88.3654) projected
  line L271 (87.7843, 88.3654) -> (98.4236, 99.0047) projected
  line L272 (54.6, 99.0047) -> (59.7861, 93.8186) projected
  line L273 (59.7861, 93.8186) -> (54.6, 99.0047) projected
  line L274 (81.1911, 93.8186) -> (59.7861, 93.8186) projected
  line L275 (59.7861, 93.8186) -> (81.1911, 93.8186) projected
  line L276 (-84.3661, -53.4337) -> (-84.3661, -85.944) projected
  line L277 (-84.3661, -53.4337) -> (-84.3661, -85.944) projected
  line L278 (-84.3661, -85.944) -> (-84.3661, -53.4337) projected
  line L279 (-84.3661, -85.944) -> (-84.3661, -53.4337) projected
  line L280 (51.0079, -101.4346) -> (42.2297, -92.6564) projected
  line L281 (42.2297, -92.6564) -> (51.0079, -101.4346) projected
  line L282 (47.4158, -105.0267) -> (35.0455, -92.6564) projected
  line L283 (35.0455, -92.6564) -> (47.4158, -105.0267) projected
  line L284 (81.1911, -89.119) -> (-81.1911, -89.119) projected
  line L285 (-81.1911, -89.119) -> (81.1911, -89.119) projected
  line L286 (-81.1911, -89.119) -> (81.1911, -89.119) projected
  line L287 (81.1911, -89.119) -> (-81.1911, -89.119) projected
  line L288 (-81.1911, 90.2812) -> (81.1911, 90.2812) projected
  arc A74 (84.3661, 87.1062) -> (81.1911, 90.2812) centre (81.1911, 87.1062) ccw projected
  line L289 (84.3661, 87.1062) -> (84.3661, 54.5958) projected
  arc A75 (84.3661, 54.5958) -> (87.5411, 51.4208) centre (87.5411, 54.5958) ccw projected
  line L290 (87.5411, 51.4208) -> (88.0954, 51.4208) projected
  arc A76 (91.2704, 48.2458) -> (88.0954, 51.4208) centre (88.0954, 48.2458) ccw projected
  line L291 (91.2704, 48.2458) -> (91.2704, -47.0837) projected
  arc A77 (88.0954, -50.2587) -> (91.2704, -47.0837) centre (88.0954, -47.0837) ccw projected
  line L292 (88.0954, -50.2587) -> (87.5411, -50.2587) projected
  arc A78 (87.5411, -50.2587) -> (84.3661, -53.4337) centre (87.5411, -53.4337) ccw projected
  line L293 (84.3661, -53.4337) -> (84.3661, -85.944) projected
  arc A79 (81.1911, -89.119) -> (84.3661, -85.944) centre (81.1911, -85.944) ccw projected
  line L294 (81.1911, -89.119) -> (-81.1911, -89.119) projected
  arc A80 (-84.3661, -85.944) -> (-81.1911, -89.119) centre (-81.1911, -85.944) ccw projected
  line L295 (-84.3661, -85.944) -> (-84.3661, -53.4337) projected
  arc A81 (-84.3661, -53.4337) -> (-87.5411, -50.2587) centre (-87.5411, -53.4337) ccw projected
  line L296 (-87.5411, -50.2587) -> (-88.0954, -50.2587) projected
  arc A82 (-91.2704, -47.0837) -> (-88.0954, -50.2587) centre (-88.0954, -47.0837) ccw projected
  line L297 (-91.2704, -47.0837) -> (-91.2704, 48.2458) projected
  arc A83 (-88.0954, 51.4208) -> (-91.2704, 48.2458) centre (-88.0954, 48.2458) ccw projected
  line L298 (-88.0954, 51.4208) -> (-87.5411, 51.4208) projected
  arc A84 (-87.5411, 51.4208) -> (-84.3661, 54.5958) centre (-87.5411, 54.5958) ccw projected
  line L299 (-84.3661, 54.5958) -> (-84.3661, 87.1062) projected
  arc A85 (-81.1911, 90.2812) -> (-84.3661, 87.1062) centre (-81.1911, 87.1062) ccw projected
  line L300 (59.7861, -92.6564) -> (51.0079, -101.4346) projected
  line L301 (51.0079, -101.4346) -> (42.2297, -92.6564) projected
  line L302 (42.2297, -92.6564) -> (59.7861, -92.6564) projected
  line L303 (35.0455, -92.6564) -> (47.4158, -105.0267) projected
  line L304 (47.4158, -105.0267) -> (25.5039, -126.9386) projected
  line L305 (25.5039, -126.9386) -> (3.5921, -105.0267) projected
  line L306 (3.5921, -105.0267) -> (15.9624, -92.6564) projected
  line L307 (15.9624, -92.6564) -> (35.0455, -92.6564) projected
  line L308 (-66.9703, -92.6564) -> (-54.6, -105.0267) projected
  line L309 (-54.6, -105.0267) -> (-76.5118, -126.9386) projected
  line L310 (-76.5118, -126.9386) -> (-98.4236, -105.0267) projected
  line L311 (-98.4236, -105.0267) -> (-84.9214, -91.5245) projected
  arc A86 (-84.9214, -91.5245) -> (-81.1911, -92.6564) centre (-81.1911, -85.944) ccw projected
  line L312 (-81.1911, -92.6564) -> (-66.9703, -92.6564) projected
  line L313 (-87.7843, -87.2033) -> (-102.0157, -101.4346) projected
  line L314 (-102.0157, -101.4346) -> (-123.9275, -79.5228) projected
  line L315 (-123.9275, -79.5228) -> (-102.0157, -57.611) projected
  line L316 (-102.0157, -57.611) -> (-87.9035, -71.7232) projected
  line L317 (-87.9035, -71.7232) -> (-87.9035, -85.944) projected
  arc A87 (-87.9035, -85.944) -> (-87.7843, -87.2033) centre (-81.1911, -85.944) ccw projected
  line L318 (-87.9035, -64.539) -> (-98.4236, -54.0189) projected
  line L319 (-98.4236, -54.0189) -> (-94.2247, -49.82) projected
  arc A88 (-94.2247, -49.82) -> (-88.0954, -53.7961) centre (-88.0954, -47.0837) ccw projected
  line L320 (-88.0954, -53.7961) -> (-87.9035, -53.7961) projected
  line L321 (-87.9035, -53.7961) -> (-87.9035, -64.539) projected
  line L322 (-94.8078, 7.789) -> (-102.0157, 0.5811) projected
  line L323 (-102.0157, 0.5811) -> (-123.9275, 22.4929) projected
  line L324 (-123.9275, 22.4929) -> (-102.0157, 44.4047) projected
  line L325 (-102.0157, 44.4047) -> (-94.8078, 37.1968) projected
  line L326 (-94.8078, 37.1968) -> (-94.8078, 7.789) projected
  line L327 (-94.8078, -43.2189) -> (-102.0157, -50.4268) projected
  line L328 (-102.0157, -50.4268) -> (-123.9275, -28.515) projected
  line L329 (-123.9275, -28.515) -> (-102.0157, -6.6031) projected
  line L330 (-102.0157, -6.6031) -> (-94.8078, -13.8111) projected
  line L331 (-94.8078, -13.8111) -> (-94.8078, -43.2189) projected
  line L332 (-94.8078, 44.381) -> (-98.4236, 47.9968) projected
  line L333 (-98.4236, 47.9968) -> (-87.9035, 58.5169) projected
  line L334 (-87.9035, 58.5169) -> (-87.9035, 54.9582) projected
  line L335 (-87.9035, 54.9582) -> (-88.0954, 54.9582) projected
  arc A89 (-88.0954, 54.9582) -> (-94.8078, 48.2458) centre (-88.0954, 48.2458) ccw projected
  line L336 (-94.8078, 48.2458) -> (-94.8078, 44.381) projected
  line L337 (-87.7843, 88.3654) -> (-98.4236, 99.0047) projected
  line L338 (-98.4236, 99.0047) -> (-76.5118, 120.9165) projected
  line L339 (-76.5118, 120.9165) -> (-54.6, 99.0047) projected
  line L340 (-54.6, 99.0047) -> (-59.7861, 93.8186) projected
  line L341 (-59.7861, 93.8186) -> (-81.1911, 93.8186) projected
  arc A90 (-81.1911, 93.8186) -> (-87.7843, 88.3654) centre (-81.1911, 87.1062) ccw projected
  line L342 (-52.6018, 93.8186) -> (-51.0079, 95.4126) projected
  line L343 (-51.0079, 95.4126) -> (-49.4139, 93.8186) projected
  line L344 (-49.4139, 93.8186) -> (-52.6018, 93.8186) projected
  line L345 (-42.2297, 93.8186) -> (-47.4158, 99.0047) projected
  line L346 (-47.4158, 99.0047) -> (-25.5039, 120.9165) projected
  line L347 (-25.5039, 120.9165) -> (-3.5921, 99.0047) projected
  line L348 (-3.5921, 99.0047) -> (-8.7782, 93.8186) projected
  line L349 (-8.7782, 93.8186) -> (-42.2297, 93.8186) projected
  line L350 (66.9703, -92.6564) -> (81.1911, -92.6564) projected
  arc A91 (81.1911, -92.6564) -> (84.9214, -91.5245) centre (81.1911, -85.944) ccw projected
  line L351 (84.9214, -91.5245) -> (98.4236, -105.0267) projected
  line L352 (98.4236, -105.0267) -> (76.5118, -126.9386) projected
  line L353 (76.5118, -126.9386) -> (54.6, -105.0267) projected
  line L354 (54.6, -105.0267) -> (66.9703, -92.6564) projected
  line L355 (-59.7861, -92.6564) -> (-42.2297, -92.6564) projected
  line L356 (-42.2297, -92.6564) -> (-51.0079, -101.4346) projected
  line L357 (-51.0079, -101.4346) -> (-59.7861, -92.6564) projected
  line L358 (-35.0455, -92.6564) -> (-15.9624, -92.6564) projected
  line L359 (-15.9624, -92.6564) -> (-3.5921, -105.0267) projected
  line L360 (-3.5921, -105.0267) -> (-25.5039, -126.9386) projected
  line L361 (-25.5039, -126.9386) -> (-47.4158, -105.0267) projected
  line L362 (-47.4158, -105.0267) -> (-35.0455, -92.6564) projected
  line L363 (-8.7782, -92.6564) -> (8.7782, -92.6564) projected
  line L364 (8.7782, -92.6564) -> (0, -101.4346) projected
  line L365 (0, -101.4346) -> (-8.7782, -92.6564) projected
  arc A92 (87.7843, -87.2033) -> (87.9035, -85.944) centre (81.1911, -85.944) ccw projected
  line L366 (87.9035, -85.944) -> (87.9035, -71.7232) projected
  line L367 (87.9035, -71.7232) -> (102.0157, -57.611) projected
  line L368 (102.0157, -57.611) -> (123.9275, -79.5228) projected
  line L369 (123.9275, -79.5228) -> (102.0157, -101.4346) projected
  line L370 (102.0157, -101.4346) -> (87.7843, -87.2033) projected
  line L371 (87.9035, -64.539) -> (87.9035, -53.7961) projected
  line L372 (87.9035, -53.7961) -> (88.0954, -53.7961) projected
  arc A93 (88.0954, -53.7961) -> (94.2247, -49.82) centre (88.0954, -47.0837) ccw projected
  line L373 (94.2247, -49.82) -> (98.4236, -54.0189) projected
  line L374 (98.4236, -54.0189) -> (87.9035, -64.539) projected
  line L375 (-94.8078, 0.6048) -> (-94.8078, -6.6269) projected
  line L376 (-94.8078, -6.6269) -> (-98.4236, -3.011) projected
  line L377 (-98.4236, -3.011) -> (-94.8078, 0.6048) projected
  line L378 (-87.9035, 81.3004) -> (-87.9035, 65.7011) projected
  line L379 (-87.9035, 65.7011) -> (-102.0157, 51.5889) projected
  line L380 (-102.0157, 51.5889) -> (-123.9275, 73.5007) projected
  line L381 (-123.9275, 73.5007) -> (-102.0157, 95.4126) projected
  line L382 (-102.0157, 95.4126) -> (-87.9035, 81.3004) projected
  line L383 (94.8078, -43.2189) -> (94.8078, -13.8111) projected
  line L384 (94.8078, -13.8111) -> (102.0157, -6.6031) projected
  line L385 (102.0157, -6.6031) -> (123.9275, -28.515) projected
  line L386 (123.9275, -28.515) -> (102.0157, -50.4268) projected
  line L387 (102.0157, -50.4268) -> (94.8078, -43.2189) projected
  line L388 (94.8078, -6.6269) -> (94.8078, 0.6048) projected
  line L389 (94.8078, 0.6048) -> (98.4236, -3.011) projected
  line L390 (98.4236, -3.011) -> (94.8078, -6.6269) projected
  line L391 (94.8078, 7.789) -> (94.8078, 37.1968) projected
  line L392 (94.8078, 37.1968) -> (102.0157, 44.4047) projected
  line L393 (102.0157, 44.4047) -> (123.9275, 22.4929) projected
  line L394 (123.9275, 22.4929) -> (102.0157, 0.5811) projected
  line L395 (102.0157, 0.5811) -> (94.8078, 7.789) projected
  line L396 (94.8078, 44.381) -> (94.8078, 48.2458) projected
  arc A94 (94.8078, 48.2458) -> (88.0954, 54.9582) centre (88.0954, 48.2458) ccw projected
  line L397 (88.0954, 54.9582) -> (87.9035, 54.9582) projected
  line L398 (87.9035, 54.9582) -> (87.9035, 58.5169) projected
  line L399 (87.9035, 58.5169) -> (98.4236, 47.9968) projected
  line L400 (98.4236, 47.9968) -> (94.8078, 44.381) projected
  line L401 (87.9035, 65.7011) -> (87.9035, 81.3004) projected
  line L402 (87.9035, 81.3004) -> (102.0157, 95.4126) projected
  line L403 (102.0157, 95.4126) -> (123.9275, 73.5007) projected
  line L404 (123.9275, 73.5007) -> (102.0157, 51.5889) projected
  line L405 (102.0157, 51.5889) -> (87.9035, 65.7011) projected
  arc A95 (87.7843, 88.3654) -> (81.1911, 93.8186) centre (81.1911, 87.1062) ccw projected
  line L406 (81.1911, 93.8186) -> (59.7861, 93.8186) projected
  line L407 (59.7861, 93.8186) -> (54.6, 99.0047) projected
  line L408 (54.6, 99.0047) -> (76.5118, 120.9165) projected
  line L409 (76.5118, 120.9165) -> (98.4236, 99.0047) projected
  line L410 (98.4236, 99.0047) -> (87.7843, 88.3654) projected
  line L411 (42.2297, 93.8186) -> (8.7782, 93.8186) projected
  line L412 (8.7782, 93.8186) -> (3.5921, 99.0047) projected
  line L413 (3.5921, 99.0047) -> (25.5039, 120.9165) projected
  line L414 (25.5039, 120.9165) -> (47.4158, 99.0047) projected
  line L415 (47.4158, 99.0047) -> (42.2297, 93.8186) projected
  line L416 (1.594, 93.8186) -> (-1.594, 93.8186) projected
  line L417 (-1.594, 93.8186) -> (0, 95.4126) projected
  line L418 (0, 95.4126) -> (1.594, 93.8186) projected
  line L419 (-311.15, -158.75) -> (-222.25, -158.75) projected
  arc A96 (-158.75, -222.25) -> (-222.25, -158.75) centre (-222.25, -222.25) ccw projected
  line L420 (-158.75, -222.25) -> (-158.75, -311.15) projected
  line L421 (-158.75, -311.15) -> (158.75, -311.15) projected
  line L422 (158.75, -311.15) -> (158.75, -222.25) projected
  arc A97 (222.25, -158.75) -> (158.75, -222.25) centre (222.25, -222.25) ccw projected
  line L423 (222.25, -158.75) -> (311.15, -158.75) projected
  line L424 (311.15, -158.75) -> (311.15, 158.75) projected
  line L425 (311.15, 158.75) -> (222.25, 158.75) projected
  arc A98 (158.75, 222.25) -> (222.25, 158.75) centre (222.25, 222.25) ccw projected
  line L426 (158.75, 222.25) -> (158.75, 311.15) projected
  line L427 (158.75, 311.15) -> (-158.75, 311.15) projected
  line L428 (-158.75, 311.15) -> (-158.75, 222.25) projected
  arc A99 (-222.25, 158.75) -> (-158.75, 222.25) centre (-222.25, 222.25) ccw projected
  line L429 (-222.25, 158.75) -> (-311.15, 158.75) projected
  line L430 (-311.15, 158.75) -> (-311.15, -158.75) projected
  circle A100 centre (-304.8, 88.9) radius 1.9939 projected
  circle A101 centre (-304.8, -133.35) radius 1.9939 projected
  circle A102 centre (0, -304.8) radius 1.9939 projected
  circle A103 centre (304.8, -133.35) radius 1.9939 projected
  circle A104 centre (304.8, 44.45) radius 1.9939 projected
  circle A105 centre (88.9, 304.8) radius 1.9939 projected
  circle A106 centre (-88.9, 304.8) radius 1.9939 projected
  circle A107 centre (-44.45, 304.8) radius 1.9939 projected
  circle A108 centre (133.35, 304.8) radius 1.9939 projected
  circle A109 centre (133.35, -304.8) radius 1.9939 projected
  circle A110 centre (-44.45, -304.8) radius 1.9939 projected
  circle A111 centre (-304.8, -88.9) radius 1.9939 projected
  circle A112 centre (-304.8, 133.35) radius 1.9939 projected
  circle A113 centre (-304.8, 44.45) radius 1.9939 projected
  circle A114 centre (-133.35, -304.8) radius 1.9939 projected
  circle A115 centre (44.45, -304.8) radius 1.9939 projected
  circle A116 centre (304.8, -88.9) radius 1.9939 projected
  circle A117 centre (304.8, 88.9) radius 1.9939 projected
  circle A118 centre (44.45, 304.8) radius 1.9939 projected
  circle A119 centre (-133.35, 304.8) radius 1.9939 projected
  circle A120 centre (0, 304.8) radius 1.9939 projected
  circle A121 centre (304.8, 133.35) radius 1.9939 projected
  circle A122 centre (304.8, -44.45) radius 1.9939 projected
  circle A123 centre (88.9, -304.8) radius 1.9939 projected